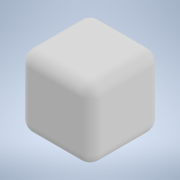
# Autodesk Inventor part: kubik
Saved by Autodesk Inventor 2022 (Build 260153000, 153)
## iProperties
Created: 2024-09-27
Part Number: kubik
Material: Типовые
Document SubType Name: Modeling
Designer: Andrey
Density: 1 g/cm^3
Appearance: По умолчанию
Author: Andrey
Autodesk Inventor part; units mm, degrees
ref_plane "YZ Plane" through (0, 0, 0) normal (1, 0, 0) x (0, 1, 0)
ref_plane "XZ Plane" through (0, 0, 0) normal (0, 1, 0) x (-1, 0, 0)
ref_plane "XY Plane" through (0, 0, 0) normal (0, 0, 1) x (1, 0, 0)
sketch "Эскиз1" plane through (0, 0, 0) normal (0, 1, 0) x (-1, 0, 0)
  line L0 (-5.25, 5.25) -> (5.25, 5.25)
  line L1 (5.25, 5.25) -> (5.25, -5.25)
  line L2 (5.25, -5.25) -> (-5.25, -5.25)
  line L3 (-5.25, -5.25) -> (-5.25, 5.25)
  line L4 (-5.25, 5.25) -> (5.25, -5.25) construction
  line L5 (5.25, 5.25) -> (-5.25, -5.25) construction
  point P0 (0, 0)
  dimension "d0" = 10.5
  dimension "d1" = 10.5
  constraints: 12 end point, 2 midpoint, 2 parallel, 1 horizontal, 1 perpendicular
  measures "d0" distance of L1.end L2.end
  measures "d1" distance of L0.end L1.end
extrude "Выдавливание1" add sketch "Эскиз1" along normal blind 10.5
fillet "Сопряжение1" radius 1.7 12 edges at (5.25, 10.5, 0) (0, 10.5, 5.25) (-5.25, 10.5, 0) (0, 10.5, -5.25) (0, 0, -5.25) (-5.25, 5.25, -5.25) (-5.25, 0, 0) (-5.25, 5.25, 5.25) (0, 0, 5.25) (5.25, 5.25, 5.25) (5.25, 5.25, -5.25) (5.25, 0, 0)
